Autodesk Inventor part; units mm, degrees
(part 2 of 3)
  spline S19 degree 4 poles (63.2685, 70.0081) (62.9924, 70.1512) (62.9774, 70.3018) (63.4893, 70.4674) (66.6514, 70.9944) (71.9063, 71.3106) (74.9329, 71.4009) (78.0798, 71.4009) (79.706, 71.3859) (80.218, 71.3859) (80.6245, 70.9643) (81.1365, 70.1662) (81.5129, 69.5639) (81.5975, 68.8428) knots 1 1 1 1 1 2 3 4 5 6 7 8 9 10 11 11 11 11 11
  line L530 (83.8243, 70.3846) -> (83.4753, 70.6213) construction
  line L531 (83.4753, 70.6213) -> (83.5043, 70.8246) construction
  line L532 (83.5043, 70.8246) -> (83.9543, 70.8826) construction
  line L533 (83.9543, 70.8826) -> (85.6239, 70.9407) construction
  line L534 (85.6239, 70.9407) -> (88.3822, 70.4181) construction
  line L535 (88.3822, 70.4181) -> (91.8016, 69.5461) construction
  line L536 (91.8016, 69.5461) -> (94.4571, 68.9806) construction
  line L537 (94.4571, 68.9806) -> (97.6535, 67.7512) construction
  line L538 (97.6535, 67.7512) -> (99.3008, 67.0382) construction
  line L539 (99.3008, 67.0382) -> (99.4975, 66.7677) construction
  line L540 (99.4975, 66.7677) -> (99.2517, 65.3908) construction
  line L541 (99.2517, 65.3908) -> (98.9566, 63.1533) construction
  line L542 (98.9566, 63.1533) -> (99.0304, 62.3911) construction
  line L543 (99.0304, 62.3911) -> (98.6616, 62.4649) construction
  line L544 (98.6616, 62.4649) -> (97.7272, 63.1041) construction
  line L545 (97.7272, 63.1041) -> (96.2766, 64.3581) construction
  line L546 (96.2766, 64.3581) -> (94.6292, 65.6121) construction
  line L547 (94.6292, 65.6121) -> (93.7194, 66.3497) construction
  line L548 (93.7194, 66.3497) -> (93.1539, 66.7185) construction
  line L549 (93.1539, 66.7185) -> (91.6786, 66.2022) construction
  line L550 (91.6786, 66.2022) -> (91.064, 64.8499) construction
  line L551 (91.064, 64.8499) -> (90.8673, 64.0139) construction
  line L552 (90.8673, 64.0139) -> (91.359, 62.9074) construction
  line L553 (91.359, 62.9074) -> (91.9491, 61.5551) construction
  line L554 (91.9491, 61.5551) -> (92.0596, 61.2579) construction
  line L555 (92.0596, 61.2579) -> (92.1675, 61.1272) construction
  spline S20 degree 4 poles (83.8243, 70.3846) (83.4753, 70.6213) (83.5043, 70.8246) (83.9543, 70.8826) (85.6239, 70.9407) (88.3822, 70.4181) (91.8016, 69.5461) (94.4571, 68.9806) (97.6535, 67.7512) (99.3008, 67.0382) (99.4975, 66.7677) (99.2517, 65.3908) (98.9566, 63.1533) (99.0304, 62.3911) (98.6616, 62.4649) (97.7272, 63.1041) (96.2766, 64.3581) (94.6292, 65.6121) (93.7194, 66.3497) (93.1539, 66.7185) (91.6786, 66.2022) (91.064, 64.8499) (90.8673, 64.0139) (91.359, 62.9074) (91.9491, 61.5551) (92.0596, 61.2579) (92.1675, 61.1272) knots 1 1 1 1 1 2 3 4 5 6 7 8 9 10 11 12 13 14 15 16 17 18 19 20 21 22 23 24 24 24 24 24
  line L556 (92.0596, 60.9567) -> (90.2836, 60.8762) construction
  line L557 (90.2836, 60.8762) -> (89.3753, 60.8573) construction
  line L558 (89.3753, 60.8573) -> (87.0288, 60.6113) construction
  line L559 (87.0288, 60.6113) -> (85.6286, 60.6491) construction
  line L560 (85.6286, 60.6491) -> (84.6446, 60.5923) construction
  line L561 (84.6446, 60.5923) -> (84.7203, 59.684) construction
  line L562 (84.7203, 59.684) -> (84.4932, 59.1921) construction
  line L563 (84.4932, 59.1921) -> (83.9066, 59.211) construction
  line L564 (83.9066, 59.211) -> (82.7523, 59.4948) construction
  line L565 (82.7523, 59.4948) -> (81.2763, 59.8733) construction
  line L566 (81.2763, 59.8733) -> (78.1729, 60.0814) construction
  line L567 (78.1729, 60.0814) -> (74.5776, 60.0625) construction
  line L568 (74.5776, 60.0625) -> (70.7362, 60.1382) construction
  line L569 (70.7362, 60.1382) -> (68.1817, 60.0625) construction
  line L570 (68.1817, 60.0625) -> (65.7974, 60.0057) construction
  line L571 (65.7974, 60.0057) -> (62.3156, 59.4759) construction
  line L572 (62.3156, 59.4759) -> (59.761, 58.7758) construction
  line L573 (59.761, 58.7758) -> (57.3956, 58.1702) construction
  line L574 (57.3956, 58.1702) -> (56.7712, 57.9053) construction
  line L575 (56.7712, 57.9053) -> (56.8847, 57.0916) construction
  line L576 (56.8847, 57.0916) -> (57.2064, 56.4104) construction
  line L577 (57.2064, 56.4104) -> (58.9284, 56.2022) construction
  line L578 (58.9284, 56.2022) -> (61.1234, 55.9373) construction
  line L579 (61.1234, 55.9373) -> (63.5266, 55.4832) construction
  line L580 (63.5266, 55.4832) -> (65.0594, 55.1047) construction
  line L581 (65.0594, 55.1047) -> (65.3354, 54.7866) construction
  spline S21 degree 4 poles (92.0596, 60.9567) (90.2836, 60.8762) (89.3753, 60.8573) (87.0288, 60.6113) (85.6286, 60.6491) (84.6446, 60.5923) (84.7203, 59.684) (84.4932, 59.1921) (83.9066, 59.211) (82.7523, 59.4948) (81.2763, 59.8733) (78.1729, 60.0814) (74.5776, 60.0625) (70.7362, 60.1382) (68.1817, 60.0625) (65.7974, 60.0057) (62.3156, 59.4759) (59.761, 58.7758) (57.3956, 58.1702) (56.7712, 57.9053) (56.8847, 57.0916) (57.2064, 56.4104) (58.9284, 56.2022) (61.1234, 55.9373) (63.5266, 55.4832) (65.0594, 55.1047) (65.3354, 54.7866) knots 1 1 1 1 1 2 3 4 5 6 7 8 9 10 11 12 13 14 15 16 17 18 19 20 21 22 23 24 24 24 24 24
  line L582 (65.4191, 54.3358) -> (65.081, 53.9607) construction
  line L583 (65.081, 53.9607) -> (63.7918, 52.863) construction
  line L584 (63.7918, 52.863) -> (62.9342, 51.842) construction
  line L585 (62.9342, 51.842) -> (61.7906, 50.5759) construction
  line L586 (61.7906, 50.5759) -> (61.0351, 49.269) construction
  line L587 (61.0351, 49.269) -> (60.2182, 48.2888) construction
  line L588 (60.2182, 48.2888) -> (59.4831, 46.5326) construction
  line L589 (59.4831, 46.5326) -> (59.1155, 45.144) construction
  line L590 (59.1155, 45.144) -> (58.6459, 43.4696) construction
  line L591 (58.6459, 43.4696) -> (58.217, 41.6113) construction
  line L592 (58.217, 41.6113) -> (58.0128, 38.9975) construction
  line L593 (58.0128, 38.9975) -> (57.9924, 37.4659) construction
  line L594 (57.9924, 37.4659) -> (57.8131, 36.3636) construction
  spline S22 degree 4 poles (65.4191, 54.3358) (65.081, 53.9607) (63.7918, 52.863) (62.9342, 51.842) (61.7906, 50.5759) (61.0351, 49.269) (60.2182, 48.2888) (59.4831, 46.5326) (59.1155, 45.144) (58.6459, 43.4696) (58.217, 41.6113) (58.0128, 38.9975) (57.9924, 37.4659) (57.8131, 36.3636) knots 1 1 1 1 1 2 3 4 5 6 7 8 9 10 11 11 11 11 11
  line L595 (8.3598, 43.6237) -> (9.8064, 44.3371) construction
  line L596 (9.8064, 44.3371) -> (11.9481, 45.3894) construction
  line L597 (11.9481, 45.3894) -> (15.3774, 46.6645) construction
  line L598 (15.3774, 46.6645) -> (20.0406, 48.2611) construction
  line L599 (20.0406, 48.2611) -> (24.339, 49.7917) construction
  line L600 (24.339, 49.7917) -> (29.2664, 51.3853) construction
  line L601 (29.2664, 51.3853) -> (32.9147, 52.5385) construction
  line L602 (32.9147, 52.5385) -> (36.626, 53.524) construction
  line L603 (36.626, 53.524) -> (38.6389, 54.174) construction
  line L604 (38.6389, 54.174) -> (40.6099, 54.174) construction
  line L605 (40.6099, 54.174) -> (43.5034, 53.2723) construction
  line L606 (43.5034, 53.2723) -> (46.2292, 52.9788) construction
  line L607 (46.2292, 52.9788) -> (48.934, 52.853) construction
  line L608 (48.934, 52.853) -> (51.5759, 52.6643) construction
  line L609 (51.5759, 52.6643) -> (52.6732, 52.6191) construction
  line L610 (52.6732, 52.6191) -> (53.2041, 52.6249) construction
  line L611 (53.2041, 52.6249) -> (53.245, 52.409) construction
  line L612 (53.245, 52.409) -> (52.8832, 51.8547) construction
  line L613 (52.8832, 51.8547) -> (51.8388, 50.6003) construction
  line L614 (51.8388, 50.6003) -> (50.5853, 48.4878) construction
  line L615 (50.5853, 48.4878) -> (49.3133, 45.3915) construction
  line L616 (49.3133, 45.3915) -> (48.2924, 42.3454) construction
  line L617 (48.2924, 42.3454) -> (47.9242, 40.2365) construction
  line L618 (47.9242, 40.2365) -> (48.192, 39.5168) construction
  line L619 (48.192, 39.5168) -> (48.8112, 38.9478) construction
  line L620 (48.8112, 38.9478) -> (48.51, 38.5126) construction
  line L621 (48.51, 38.5126) -> (48.0915, 37.3578) construction
  line L622 (48.0915, 37.3578) -> (48.0078, 36.3535) construction
  line L623 (48.0078, 36.3535) -> (48.7108, 34.6129) construction
  line L624 (48.7108, 34.6129) -> (49.6313, 32.4036) construction
  line L625 (49.6313, 32.4036) -> (50.8364, 30.0939) construction
  line L626 (50.8364, 30.0939) -> (52.008, 28.6546) construction
  line L627 (52.008, 28.6546) -> (54.3177, 26.0771) construction
  line L628 (54.3177, 26.0771) -> (55.9411, 24.6879) construction
  line L629 (55.9411, 24.6879) -> (57.2466, 24.1858) construction
  line L630 (57.2466, 24.1858) -> (57.7487, 24.3364) construction
  line L631 (57.7487, 24.3364) -> (58.4851, 24.4201) construction
  line L632 (58.4851, 24.4201) -> (58.865, 24.189) construction
  line L633 (58.865, 24.189) -> (58.95, 23.1685) construction
  line L634 (58.95, 23.1685) -> (59.8855, 22.2898) construction
  line L635 (59.8855, 22.2898) -> (62.465, 21.2409) construction
  line L636 (62.465, 21.2409) -> (65.5265, 20.5889) construction
  line L637 (65.5265, 20.5889) -> (70.7139, 20.0504) construction
  line L638 (70.7139, 20.0504) -> (74.4557, 19.937) construction
  line L639 (74.4557, 19.937) -> (76.8368, 20.0504) construction
  line L640 (76.8368, 20.0504) -> (78.3912, 20.0214) construction
  line L641 (78.3912, 20.0214) -> (78.6619, 19.922) construction
  spline S23 degree 4 poles (8.3598, 43.6237) (9.8064, 44.3371) (11.9481, 45.3894) (15.3774, 46.6645) (20.0406, 48.2611) (24.339, 49.7917) (29.2664, 51.3853) (32.9147, 52.5385) (36.626, 53.524) (38.6389, 54.174) (40.6099, 54.174) (43.5034, 53.2723) (46.2292, 52.9788) (48.934, 52.853) (51.5759, 52.6643) (52.6732, 52.6191) (53.2041, 52.6249) (53.245, 52.409) (52.8832, 51.8547) (51.8388, 50.6003) (50.5853, 48.4878) (49.3133, 45.3915) (48.2924, 42.3454) (47.9242, 40.2365) (48.192, 39.5168) (48.8112, 38.9478) (48.51, 38.5126) (48.0915, 37.3578) (48.0078, 36.3535) (48.7108, 34.6129) (49.6313, 32.4036) (50.8364, 30.0939) (52.008, 28.6546) (54.3177, 26.0771) (55.9411, 24.6879) (57.2466, 24.1858) (57.7487, 24.3364) (58.4851, 24.4201) (58.865, 24.189) (58.95, 23.1685) (59.8855, 22.2898) (62.465, 21.2409) (65.5265, 20.5889) (70.7139, 20.0504) (74.4557, 19.937) (76.8368, 20.0504) (78.3912, 20.0214) (78.6619, 19.922) knots 1 1 1 1 1 2 3 4 5 6 7 8 9 10 11 12 13 14 15 16 17 18 19 20 21 22 23 24 25 26 27 28 29 30 31 32 33 34 35 36 37 38 39 40 41 42 43 44 45 45 45 45 45
  line L642 (65.081, 28.397) -> (65.0019, 29.199) construction
  line L643 (65.0019, 29.199) -> (65.2705, 30.0048) construction
  line L644 (65.2705, 30.0048) -> (65.4415, 30.9327) construction
  line L645 (65.4415, 30.9327) -> (64.9043, 31.9338) construction
  line L646 (64.9043, 31.9338) -> (64.831, 33.4477) construction
  line L647 (64.831, 33.4477) -> (64.8066, 36.0849) construction
  line L648 (64.8066, 36.0849) -> (65.2217, 38.3313) construction
  line L649 (65.2217, 38.3313) -> (65.881, 39.4545) construction
  line L650 (65.881, 39.4545) -> (66.0763, 40.0162) construction
  line L651 (66.0763, 40.0162) -> (65.9054, 40.1383) construction
  line L652 (65.9054, 40.1383) -> (65.5265, 40.0607) construction
  line L653 (65.5265, 40.0607) -> (65.4932, 40.0607) construction
  spline S24 degree 4 poles (65.081, 28.397) (65.0019, 29.199) (65.2705, 30.0048) (65.4415, 30.9327) (64.9043, 31.9338) (64.831, 33.4477) (64.8066, 36.0849) (65.2217, 38.3313) (65.881, 39.4545) (66.0763, 40.0162) (65.9054, 40.1383) (65.5265, 40.0607) (65.4932, 40.0607) knots 1 1 1 1 1 2 3 4 5 6 7 8 9 10 10 10 10 10
  line L654 (52.8179, 63.6057) -> (51.2391, 63.3355) construction
  line L655 (51.2391, 63.3355) -> (49.1343, 62.8712) construction
  line L656 (49.1343, 62.8712) -> (46.2247, 62.6546) construction
  line L657 (46.2247, 62.6546) -> (43.9342, 63.676) construction
  line L658 (43.9342, 63.676) -> (42.4794, 64.1713) construction
  line L659 (42.4794, 64.1713) -> (43.7175, 63.0879) construction
  line L660 (43.7175, 63.0879) -> (46.2557, 61.726) construction
  line L661 (46.2557, 61.726) -> (47.0295, 61.3545) construction
  line L662 (47.0295, 61.3545) -> (49.2581, 61.6641) construction
  line L663 (49.2581, 61.6641) -> (51.6725, 61.695) construction
  line L664 (51.6725, 61.695) -> (53.5606, 62.1903) construction
  line L665 (53.5606, 62.1903) -> (54.5202, 62.9022) construction
  line L666 (54.5202, 62.9022) -> (58.2346, 64.7594) construction
  line L667 (58.2346, 64.7594) -> (59.256, 65.3475) construction
  line L668 (59.256, 65.3475) -> (58.5558, 65.9056) construction
  line L669 (58.5558, 65.9056) -> (57.07, 66.4008) construction
  line L670 (57.07, 66.4008) -> (54.8104, 66.8342) construction
  line L671 (54.8104, 66.8342) -> (53.1699, 66.8961) construction
  line L672 (53.1699, 66.8961) -> (51.158, 66.927) construction
  line L673 (51.158, 66.927) -> (49.3317, 66.8342) construction
  line L674 (49.3317, 66.8342) -> (48.7746, 66.6794) construction
  line L675 (48.7746, 66.6794) -> (49.7935, 66.0783) construction
  line L676 (49.7935, 66.0783) -> (50.5932, 66.0134) construction
  line L677 (50.5932, 66.0134) -> (51.2955, 65.9403) construction
  line L678 (51.2955, 65.9403) -> (51.6297, 65.9403) construction
  spline S25 degree 4 poles (52.8179, 63.6057) (51.2391, 63.3355) (49.1343, 62.8712) (46.2247, 62.6546) (43.9342, 63.676) (42.4794, 64.1713) (43.7175, 63.0879) (46.2557, 61.726) (47.0295, 61.3545) (49.2581, 61.6641) (51.6725, 61.695) (53.5606, 62.1903) (54.5202, 62.9022) (58.2346, 64.7594) (59.256, 65.3475) (58.5558, 65.9056) (57.07, 66.4008) (54.8104, 66.8342) (53.1699, 66.8961) (51.158, 66.927) (49.3317, 66.8342) (48.7746, 66.6794) (49.7935, 66.0783) (50.5932, 66.0134) (51.2955, 65.9403) (51.6297, 65.9403) knots 1 1 1 1 1 2 3 4 5 6 7 8 9 10 11 12 13 14 15 16 17 18 19 20 21 22 23 23 23 23 23
  line L679 (66.9113, 53.2103) -> (66.1589, 52.2511) construction
  line L680 (66.1589, 52.2511) -> (64.5343, 50.6524) construction
  line L681 (64.5343, 50.6524) -> (62.9548, 48.7893) construction
  line L682 (62.9548, 48.7893) -> (61.517, 46.5415) construction
  line L683 (61.517, 46.5415) -> (60.8892, 45.2657) construction
  line L684 (60.8892, 45.2657) -> (60.8082, 44.1924) construction
  line L685 (60.8082, 44.1924) -> (61.1322, 44.3342) construction
  line L686 (61.1322, 44.3342) -> (61.4562, 44.6987) construction
  line L687 (61.4562, 44.6987) -> (62.2865, 45.9745) construction
  line L688 (62.2865, 45.9745) -> (63.6028, 47.6958) construction
  line L689 (63.6028, 47.6958) -> (65.1014, 49.1538) construction
  line L690 (65.1014, 49.1538) -> (66.9644, 50.7739) construction
  line L691 (66.9644, 50.7739) -> (69.273, 52.3534) construction
  line L692 (69.273, 52.3534) -> (70.5083, 53.1432) construction
  line L693 (70.5083, 53.1432) -> (72.0878, 53.6292) construction
  line L694 (72.0878, 53.6292) -> (72.7359, 54.095) construction
  line L695 (72.7359, 54.095) -> (71.9056, 54.3988) construction
  line L696 (71.9056, 54.3988) -> (70.002, 55.067) construction
  line L697 (70.002, 55.067) -> (68.9895, 55.5935) construction
  line L698 (68.9895, 55.5935) -> (68.6524, 55.7505) construction
  line L699 (68.6524, 55.7505) -> (68.4709, 55.5789) construction
  spline S26 degree 4 poles (66.9113, 53.2103) (66.1589, 52.2511) (64.5343, 50.6524) (62.9548, 48.7893) (61.517, 46.5415) (60.8892, 45.2657) (60.8082, 44.1924) (61.1322, 44.3342) (61.4562, 44.6987) (62.2865, 45.9745) (63.6028, 47.6958) (65.1014, 49.1538) (66.9644, 50.7739) (69.273, 52.3534) (70.5083, 53.1432) (72.0878, 53.6292) (72.7359, 54.095) (71.9056, 54.3988) (70.002, 55.067) (68.9895, 55.5935) (68.6524, 55.7505) (68.4709, 55.5789) knots 1 1 1 1 1 2 3 4 5 6 7 8 9 10 11 12 13 14 15 16 17 18 19 19 19 19 19
  line L700 (66.3059, 56.3646) -> (65.6237, 56.9327) construction
  line L701 (65.6237, 56.9327) -> (64.7343, 56.992) construction
  line L702 (64.7343, 56.992) -> (64.1414, 57.1698) construction
  line L703 (64.1414, 57.1698) -> (64.3192, 57.5256) construction
  line L704 (64.3192, 57.5256) -> (65.3074, 57.7627) construction
  line L705 (65.3074, 57.7627) -> (67.8965, 58.0592) construction
  line L706 (67.8965, 58.0592) -> (72.9955, 58.2568) construction
  line L707 (72.9955, 58.2568) -> (78.8851, 58.158) construction
  line L708 (78.8851, 58.158) -> (82.6204, 57.5058) construction
  line L709 (82.6204, 57.5058) -> (87.0277, 56.7548) construction
  line L710 (87.0277, 56.7548) -> (91.5734, 55.1935) construction
  line L711 (91.5734, 55.1935) -> (95.5261, 53.2369) construction
  line L712 (95.5261, 53.2369) -> (94.9728, 53.1776) construction
  line L713 (94.9728, 53.1776) -> (90.3283, 54.7389) construction
  line L714 (90.3283, 54.7389) -> (86.0593, 55.905) construction
  line L715 (86.0593, 55.905) -> (83.747, 56.4979) construction
  line L716 (83.747, 56.4979) -> (81.8694, 56.4583) construction
  line L717 (81.8694, 56.4583) -> (81.1777, 56.5572) construction
  line L718 (81.1777, 56.5572) -> (80.6836, 57.071) construction
  line L719 (80.6836, 57.071) -> (79.7942, 57.4465) construction
  line L720 (79.7942, 57.4465) -> (75.9008, 57.5849) construction
  line L721 (75.9008, 57.5849) -> (72.5212, 57.5849) construction
  line L722 (72.5212, 57.5849) -> (68.9044, 57.5453) construction
  line L723 (68.9044, 57.5453) -> (68.2522, 57.2884) construction
  line L724 (68.2522, 57.2884) -> (68.2522, 56.6362) construction
  line L725 (68.2522, 56.6362) -> (68.0022, 56.4202) construction
  line L726 (68.0022, 56.4202) -> (67.7877, 56.3707) construction
  line L727 (67.7877, 56.3707) -> (67.6792, 56.3575) construction
  spline S27 degree 4 poles (66.3059, 56.3646) (65.6237, 56.9327) (64.7343, 56.992) (64.1414, 57.1698) (64.3192, 57.5256) (65.3074, 57.7627) (67.8965, 58.0592) (72.9955, 58.2568) (78.8851, 58.158) (82.6204, 57.5058) (87.0277, 56.7548) (91.5734, 55.1935) (95.5261, 53.2369) (94.9728, 53.1776) (90.3283, 54.7389) (86.0593, 55.905) (83.747, 56.4979) (81.8694, 56.4583) (81.1777, 56.5572) (80.6836, 57.071) (79.7942, 57.4465) (75.9008, 57.5849) (72.5212, 57.5849) (68.9044, 57.5453) (68.2522, 57.2884) (68.2522, 56.6362) (68.0022, 56.4202) (67.7877, 56.3707) (67.6792, 56.3575) knots 1 1 1 1 1 2 3 4 5 6 7 8 9 10 11 12 13 14 15 16 17 18 19 20 21 22 23 24 25 26 26 26 26 26
  line L728 (83.5333, 54.3147) -> (83.6608, 54.5518) construction
  line L729 (83.6608, 54.5518) -> (84.3663, 54.6016) construction
  line L730 (84.3663, 54.6016) -> (85.7855, 54.1285) construction
  line L731 (85.7855, 54.1285) -> (87.4123, 53.6804) construction
  line L732 (87.4123, 53.6804) -> (88.9477, 53.2737) construction
  line L733 (88.9477, 53.2737) -> (89.7196, 53.0164) construction
  line L734 (89.7196, 53.0164) -> (88.8066, 52.9002) construction
  line L735 (88.8066, 52.9002) -> (87.3625, 52.8089) construction
  line L736 (87.3625, 52.8089) -> (86.3831, 52.3939) construction
  line L737 (86.3831, 52.3939) -> (85.4535, 52.2445) construction
  line L738 (85.4535, 52.2445) -> (84.1754, 51.788) construction
  line L739 (84.1754, 51.788) -> (83.3288, 51.6718) construction
  line L740 (83.3288, 51.6718) -> (82.4823, 51.6635) construction
  line L741 (82.4823, 51.6635) -> (82.1171, 51.2818) construction
  line L742 (82.1171, 51.2818) -> (81.6357, 51.3316) construction
  line L743 (81.6357, 51.3316) -> (81.0962, 51.6303) construction
  line L744 (81.0962, 51.6303) -> (80.7974, 51.871) construction
  line L745 (80.7974, 51.871) -> (80.5485, 52.2362) construction
  line L746 (80.5485, 52.2362) -> (80.3892, 52.409) construction
  spline S28 degree 4 poles (83.5333, 54.3147) (83.6608, 54.5518) (84.3663, 54.6016) (85.7855, 54.1285) (87.4123, 53.6804) (88.9477, 53.2737) (89.7196, 53.0164) (88.8066, 52.9002) (87.3625, 52.8089) (86.3831, 52.3939) (85.4535, 52.2445) (84.1754, 51.788) (83.3288, 51.6718) (82.4823, 51.6635) (82.1171, 51.2818) (81.6357, 51.3316) (81.0962, 51.6303) (80.7974, 51.871) (80.5485, 52.2362) (80.3892, 52.409) knots 1 1 1 1 1 2 3 4 5 6 7 8 9 10 11 12 13 14 15 16 17 17 17 17 17
  line L747 (80.6729, 54.336) -> (80.4498, 54.7426) construction
  line L748 (80.4498, 54.7426) -> (79.8635, 55.2788) construction
  line L749 (79.8635, 55.2788) -> (79.6776, 55.4718) construction
  line L750 (79.6776, 55.4718) -> (79.0985, 55.6077) construction
  line L751 (79.0985, 55.6077) -> (77.8903, 55.6148) construction
  line L752 (77.8903, 55.6148) -> (76.153, 55.6506) construction
  line L753 (76.153, 55.6506) -> (75.5239, 55.6434) construction
  line L754 (75.5239, 55.6434) -> (75.3094, 55.5362) construction
  line L755 (75.3094, 55.5362) -> (75.3094, 55.3431) construction
  line L756 (75.3094, 55.3431) -> (75.8885, 55.0429) construction
  line L757 (75.8885, 55.0429) -> (76.5176, 54.6854) construction
  line L758 (76.5176, 54.6854) -> (76.9823, 54.0777) construction
  line L759 (76.9823, 54.0777) -> (76.6606, 53.6487) construction
  line L760 (76.6606, 53.6487) -> (76.1101, 53.0053) construction
  line L761 (76.1101, 53.0053) -> (75.3594, 52.655) construction
  line L762 (75.3594, 52.655) -> (73.1404, 52.0547) construction
  line L763 (73.1404, 52.0547) -> (70.3924, 50.6397) construction
  line L764 (70.3924, 50.6397) -> (66.824, 47.9942) construction
  line L765 (66.824, 47.9942) -> (64.9783, 46.292) construction
  line L766 (64.9783, 46.292) -> (63.4812, 44.5283) construction
  line L767 (63.4812, 44.5283) -> (62.4353, 42.8262) construction
  line L768 (62.4353, 42.8262) -> (61.1023, 39.955) construction
  line L769 (61.1023, 39.955) -> (60.3435, 38.0683) construction
  line L770 (60.3435, 38.0683) -> (60.323, 36.6943) construction
  line L771 (60.323, 36.6943) -> (60.323, 36.2863) construction
  spline S29 degree 4 poles (80.6729, 54.336) (80.4498, 54.7426) (79.8635, 55.2788) (79.6776, 55.4718) (79.0985, 55.6077) (77.8903, 55.6148) (76.153, 55.6506) (75.5239, 55.6434) (75.3094, 55.5362) (75.3094, 55.3431) (75.8885, 55.0429) (76.5176, 54.6854) (76.9823, 54.0777) (76.6606, 53.6487) (76.1101, 53.0053) (75.3594, 52.655) (73.1404, 52.0547) (70.3924, 50.6397) (66.824, 47.9942) (64.9783, 46.292) (63.4812, 44.5283) (62.4353, 42.8262) (61.1023, 39.955) (60.3435, 38.0683) (60.323, 36.6943) (60.323, 36.2863) knots 1 1 1 1 1 2 3 4 5 6 7 8 9 10 11 12 13 14 15 16 17 18 19 20 21 22 23 23 23 23 23
  line L772 (94.0312, 61.726) -> (93.7051, 62.2473) construction
  line L773 (93.7051, 62.2473) -> (93.1799, 63.181) construction
  line L774 (93.1799, 63.181) -> (93.1799, 63.6645) construction
  line L775 (93.1799, 63.6645) -> (93.3716, 63.8229) construction
  line L776 (93.3716, 63.8229) -> (93.7884, 63.5811) construction
  line L777 (93.7884, 63.5811) -> (94.7138, 62.9726) construction
  line L778 (94.7138, 62.9726) -> (95.7475, 62.1889) construction
  line L779 (95.7475, 62.1889) -> (97.198, 61.1469) construction
  line L780 (97.198, 61.1469) -> (97.9081, 60.597) construction
  spline S30 degree 4 poles (94.0312, 61.726) (93.7051, 62.2473) (93.1799, 63.181) (93.1799, 63.6645) (93.3716, 63.8229) (93.7884, 63.5811) (94.7138, 62.9726) (95.7475, 62.1889) (97.198, 61.1469) (97.9081, 60.597) knots 1 1 1 1 1 2 3 4 5 6 7 7 7 7 7
  line L781 (92.326, 59.0061) -> (91.721, 59.1295) construction
  line L782 (91.721, 59.1295) -> (90.1871, 59.2295) construction
  line L783 (90.1871, 59.2295) -> (89.1701, 59.2545) construction
  line L784 (89.1701, 59.2545) -> (88.1864, 59.2295) construction
  line L785 (88.1864, 59.2295) -> (87.9697, 58.9461) construction
  line L786 (87.9697, 58.9461) -> (87.9697, 58.6627) construction
  line L787 (87.9697, 58.6627) -> (87.9863, 58.4376) construction
  line L788 (87.9863, 58.4376) -> (88.4448, 58.1208) construction
  line L789 (88.4448, 58.1208) -> (90.5289, 57.5039) construction
  line L790 (90.5289, 57.5039) -> (92.513, 56.7286) construction
  line L791 (92.513, 56.7286) -> (95.2528, 55.6483) construction
  line L792 (95.2528, 55.6483) -> (98.4333, 53.807) construction
  line L793 (98.4333, 53.807) -> (102.1876, 51.6787) construction
  line L794 (102.1876, 51.6787) -> (103.8615, 50.0766) construction
  line L795 (103.8615, 50.0766) -> (105.1289, 49.3113) construction
  line L796 (105.1289, 49.3113) -> (106.0551, 49.0264) construction
  spline S31 degree 4 poles (92.326, 59.0061) (91.721, 59.1295) (90.1871, 59.2295) (89.1701, 59.2545) (88.1864, 59.2295) (87.9697, 58.9461) (87.9697, 58.6627) (87.9863, 58.4376) (88.4448, 58.1208) (90.5289, 57.5039) (92.513, 56.7286) (95.2528, 55.6483) (98.4333, 53.807) (102.1876, 51.6787) (103.8615, 50.0766) (105.1289, 49.3113) (106.0551, 49.0264) knots 1 1 1 1 1 2 3 4 5 6 7 8 9 10 11 12 13 14 14 14 14 14
  line L797 (104.2741, 46.5328) -> (103.7785, 46.9222) construction
  line L798 (103.7785, 46.9222) -> (102.9329, 47.282) construction
  line L799 (102.9329, 47.282) -> (102.3571, 47.309) construction
  line L800 (102.3571, 47.309) -> (101.6014, 47.291) construction
  line L801 (101.6014, 47.291) -> (101.4395, 47.0571) construction
  line L802 (101.4395, 47.0571) -> (100.9627, 46.6163) construction
  line L803 (100.9627, 46.6163) -> (99.9012, 46.0315) construction
  line L804 (99.9012, 46.0315) -> (99.0106, 45.6177) construction
  line L805 (99.0106, 45.6177) -> (97.931, 45.6537) construction
  line L806 (97.931, 45.6537) -> (96.6626, 45.9056) construction
  line L807 (96.6626, 45.9056) -> (95.61, 46.1305) construction
  line L808 (95.61, 46.1305) -> (94.3955, 46.2834) construction
  line L809 (94.3955, 46.2834) -> (93.2081, 46.5533) construction
  line L810 (93.2081, 46.5533) -> (92.3714, 46.5983) construction
  line L811 (92.3714, 46.5983) -> (91.9396, 46.6703) construction
  line L812 (91.9396, 46.6703) -> (91.5977, 46.4094) construction
  line L813 (91.5977, 46.4094) -> (91.022, 45.7707) construction
  line L814 (91.022, 45.7707) -> (90.5182, 45.2399) construction
  line L815 (90.5182, 45.2399) -> (90.0144, 44.7001) construction
  line L816 (90.0144, 44.7001) -> (89.4837, 44.3583) construction
  line L817 (89.4837, 44.3583) -> (88.638, 43.9624) construction
  line L818 (88.638, 43.9624) -> (88.0803, 43.9354) construction
  line L819 (88.0803, 43.9354) -> (87.5135, 43.9264) construction
  line L820 (87.5135, 43.9264) -> (87.0997, 43.8995) construction
  line L821 (87.0997, 43.8995) -> (86.7938, 43.5036) construction
  line L822 (86.7938, 43.5036) -> (86.2181, 42.721) construction
  line L823 (86.2181, 42.721) -> (85.9932, 42.2262) construction
  line L824 (85.9932, 42.2262) -> (85.5434, 41.6684) construction
  line L825 (85.5434, 41.6684) -> (85.1295, 41.2906) construction
  line L826 (85.1295, 41.2906) -> (84.3829, 40.9127) construction
  line L827 (84.3829, 40.9127) -> (83.3521, 40.3324) construction
  line L828 (83.3521, 40.3324) -> (82.4075, 39.1897) construction
  line L829 (82.4075, 39.1897) -> (81.8437, 38.1536) construction
  line L830 (81.8437, 38.1536) -> (81.4323, 37.2699) construction
  line L831 (81.4323, 37.2699) -> (81.4476, 36.3709) construction
  line L832 (81.4476, 36.3709) -> (81.3866, 35.6396) construction
  line L833 (81.3866, 35.6396) -> (81.6761, 35.1215) construction
  line L834 (81.6761, 35.1215) -> (81.8894, 34.7558) construction
  line L835 (81.8894, 34.7558) -> (82.3618, 34.0093) construction
  line L836 (82.3618, 34.0093) -> (83.0626, 33.1103) construction
  line L837 (83.0626, 33.1103) -> (83.2536, 32.9024) construction
  spline S32 degree 4 poles (104.2741, 46.5328) (103.7785, 46.9222) (102.9329, 47.282) (102.3571, 47.309) (101.6014, 47.291) (101.4395, 47.0571) (100.9627, 46.6163) (99.9012, 46.0315) (99.0106, 45.6177) (97.931, 45.6537) (96.6626, 45.9056) (95.61, 46.1305) (94.3955, 46.2834) (93.2081, 46.5533) (92.3714, 46.5983) (91.9396, 46.6703) (91.5977, 46.4094) (91.022, 45.7707) (90.5182, 45.2399) (90.0144, 44.7001) (89.4837, 44.3583) (88.638, 43.9624) (88.0803, 43.9354) (87.5135, 43.9264) (87.0997, 43.8995) (86.7938, 43.5036) (86.2181, 42.721) (85.9932, 42.2262) (85.5434, 41.6684) (85.1295, 41.2906) (84.3829, 40.9127) (83.3521, 40.3324) (82.4075, 39.1897) (81.8437, 38.1536) (81.4323, 37.2699) (81.4476, 36.3709) (81.3866, 35.6396) (81.6761, 35.1215) (81.8894, 34.7558) (82.3618, 34.0093) (83.0626, 33.1103) (83.2536, 32.9024) knots 1 1 1 1 1 2 3 4 5 6 7 8 9 10 11 12 13 14 15 16 17 18 19 20 21 22 23 24 25 26 27 28 29 30 31 32 33 34 35 36 37 38 39 39 39 39 39
  line L838 (65.9903, 42.721) -> (66.2881, 42.6424) construction
  line L839 (66.2881, 42.6424) -> (67.6606, 42.7681) construction
  line L840 (67.6606, 42.7681) -> (68.6873, 43.3757) construction
  line L841 (68.6873, 43.3757) -> (70.2797, 45.0101) construction
  line L842 (70.2797, 45.0101) -> (71.9035, 46.2672) construction
  line L843 (71.9035, 46.2672) -> (72.9093, 46.8958) construction
  line L844 (72.9093, 46.8958) -> (75.057, 48.132) construction
  line L845 (75.057, 48.132) -> (76.157, 48.9702) construction
  line L846 (76.157, 48.9702) -> (77.7285, 49.7454) construction
  line L847 (77.7285, 49.7454) -> (78.7656, 50.0597) construction
  line L848 (78.7656, 50.0597) -> (78.9434, 50.2021) construction
  spline S33 degree 4 poles (65.9903, 42.721) (66.2881, 42.6424) (67.6606, 42.7681) (68.6873, 43.3757) (70.2797, 45.0101) (71.9035, 46.2672) (72.9093, 46.8958) (75.057, 48.132) (76.157, 48.9702) (77.7285, 49.7454) (78.7656, 50.0597) (78.9434, 50.2021) knots 1 1 1 1 1 2 3 4 5 6 7 8 9 9 9 9 9
  line L849 (83.6268, 31.2422) -> (83.1411, 31.1284) construction
  line L850 (83.1411, 31.1284) -> (82.0253, 31.3729) construction
  line L851 (82.0253, 31.3729) -> (81.2611, 32.3664) construction
  line L852 (81.2611, 32.3664) -> (80.3898, 33.9101) construction
  line L853 (80.3898, 33.9101) -> (79.5951, 35.729) construction
  line L854 (79.5951, 35.729) -> (79.702, 36.967) construction
  line L855 (79.702, 36.967) -> (79.8855, 37.6854) construction
  line L856 (79.8855, 37.6854) -> (80.5427, 39.382) construction
  line L857 (80.5427, 39.382) -> (81.4292, 40.6965) construction
  line L858 (81.4292, 40.6965) -> (82.0864, 41.1397) construction
  line L859 (82.0864, 41.1397) -> (82.4227, 41.7969) construction
  line L860 (82.4227, 41.7969) -> (82.1934, 41.9192) construction
  line L861 (82.1934, 41.9192) -> (81.796, 41.7664) construction
  line L862 (81.796, 41.7664) -> (80.7567, 40.8799) construction
  line L863 (80.7567, 40.8799) -> (79.8702, 39.5501) construction
  line L864 (79.8702, 39.5501) -> (79.0907, 37.9911) construction
  line L865 (79.0907, 37.9911) -> (78.9073, 36.3251) construction
  line L866 (78.9073, 36.3251) -> (79.702, 33.849) construction
  line L867 (79.702, 33.849) -> (80.0994, 33.0084) construction
  line L868 (80.0994, 33.0084) -> (80.879, 31.5563) construction
  line L869 (80.879, 31.5563) -> (82.117, 30.2266) construction
  line L870 (82.117, 30.2266) -> (84.0428, 28.7593) construction
  line L871 (84.0428, 28.7593) -> (84.7918, 28.3619) construction
  line L872 (84.7918, 28.3619) -> (84.9829, 28.4041) construction
  spline S34 degree 4 poles (83.6268, 31.2422) (83.1411, 31.1284) (82.0253, 31.3729) (81.2611, 32.3664) (80.3898, 33.9101) (79.5951, 35.729) (79.702, 36.967) (79.8855, 37.6854) (80.5427, 39.382) (81.4292, 40.6965) (82.0864, 41.1397) (82.4227, 41.7969) (82.1934, 41.9192) (81.796, 41.7664) (80.7567, 40.8799) (79.8702, 39.5501) (79.0907, 37.9911) (78.9073, 36.3251) (79.702, 33.849) (80.0994, 33.0084) (80.879, 31.5563) (82.117, 30.2266) (84.0428, 28.7593) (84.7918, 28.3619) (84.9829, 28.4041) knots 1 1 1 1 1 2 3 4 5 6 7 8 9 10 11 12 13 14 15 16 17 18 19 20 21 22 22 22 22 22
  line L873 (85.2963, 26.5309) -> (84.6565, 26.5488) construction
  line L874 (84.6565, 26.5488) -> (83.5658, 27.0287) construction
  line L875 (83.5658, 27.0287) -> (81.6171, 28.6284) construction
  line L876 (81.6171, 28.6284) -> (79.6392, 30.7372) construction
  line L877 (79.6392, 30.7372) -> (79.1738, 31.4789) construction
  line L878 (79.1738, 31.4789) -> (78.1704, 33.5585) construction
  line L879 (78.1704, 33.5585) -> (77.5014, 34.911) construction
  line L880 (77.5014, 34.911) -> (77.3851, 36.7289) construction
  line L881 (77.3851, 36.7289) -> (77.5887, 38.8085) construction
  line L882 (77.5887, 38.8085) -> (78.0686, 40.1465) construction
  line L883 (78.0686, 40.1465) -> (79.1738, 41.6153) construction
  line L884 (79.1738, 41.6153) -> (80.3373, 42.4297) construction
  line L885 (80.3373, 42.4297) -> (81.4716, 43.3895) construction
  line L886 (81.4716, 43.3895) -> (83.7258, 44.3639) construction
  line L887 (83.7258, 44.3639) -> (85.8054, 45.1638) construction
  line L888 (85.8054, 45.1638) -> (87.9723, 45.6146) construction
  line L889 (87.9723, 45.6146) -> (88.2486, 45.8473) construction
  line L890 (88.2486, 45.8473) -> (88.1759, 46.0509) construction
  line L891 (88.1759, 46.0509) -> (87.6669, 46.1818) construction
  line L892 (87.6669, 46.1818) -> (86.5326, 46.0364) construction
  line L893 (86.5326, 46.0364) -> (83.7258, 45.2365) construction
  line L894 (83.7258, 45.2365) -> (81.1808, 43.9713) construction
  line L895 (81.1808, 43.9713) -> (79.1448, 42.6333) construction
  line L896 (79.1448, 42.6333) -> (77.865, 40.9172) construction
  line L897 (77.865, 40.9172) -> (77.036, 38.8521) construction
  line L898 (77.036, 38.8521) -> (76.6143, 36.1035) construction
  line L899 (76.6143, 36.1035) -> (76.687, 35.1291) construction
  line L900 (76.687, 35.1291) -> (77.2396, 33.6312) construction
  line L901 (77.2396, 33.6312) -> (78.4467, 31.5807) construction
  line L902 (78.4467, 31.5807) -> (79.9446, 29.5592) construction
  line L903 (79.9446, 29.5592) -> (82.2569, 27.2759) construction
  line L904 (82.2569, 27.2759) -> (85.5291, 25.1672) construction
  line L905 (85.5291, 25.1672) -> (88.1323, 23.4657) construction
  line L906 (88.1323, 23.4657) -> (88.8449, 23.3057) construction
  line L907 (88.8449, 23.3057) -> (89.6448, 23.9311) construction
  line L908 (89.6448, 23.9311) -> (89.8629, 24.4692) construction
  line L909 (89.8629, 24.4692) -> (89.5284, 25.0654) construction
  line L910 (89.5284, 25.0654) -> (89.1212, 25.9235) construction
  line L911 (89.1212, 25.9235) -> (88.7286, 27.3777) construction
  line L912 (88.7286, 27.3777) -> (89.034, 28.803) construction
  line L913 (89.034, 28.803) -> (89.543, 30.8826) construction
  line L914 (89.543, 30.8826) -> (92.052, 33.5775) construction
  line L915 (92.052, 33.5775) -> (94.4542, 35.9091) construction
  line L916 (94.4542, 35.9091) -> (96.2912, 37.1102) construction
  line L917 (96.2912, 37.1102) -> (97.9163, 38.382) construction
  line L918 (97.9163, 38.382) -> (98.9018, 39.2124) construction
  line L919 (98.9018, 39.2124) -> (98.9804, 39.5663) construction
  line L920 (98.9804, 39.5663) -> (98.4496, 39.6253) construction
  line L921 (98.4496, 39.6253) -> (97.7088, 39.6605) construction
  spline S35 degree 4 poles (85.2963, 26.5309) (84.6565, 26.5488) (83.5658, 27.0287) (81.6171, 28.6284) (79.6392, 30.7372) (79.1738, 31.4789) (78.1704, 33.5585) (77.5014, 34.911) (77.3851, 36.7289) (77.5887, 38.8085) (78.0686, 40.1465) (79.1738, 41.6153) (80.3373, 42.4297) (81.4716, 43.3895) (83.7258, 44.3639) (85.8054, 45.1638) (87.9723, 45.6146) (88.2486, 45.8473) (88.1759, 46.0509) (87.6669, 46.1818) (86.5326, 46.0364) (83.7258, 45.2365) (81.1808, 43.9713) (79.1448, 42.6333) (77.865, 40.9172) (77.036, 38.8521) (76.6143, 36.1035) (76.687, 35.1291) (77.2396, 33.6312) (78.4467, 31.5807) (79.9446, 29.5592) (82.2569, 27.2759) (85.5291, 25.1672) (88.1323, 23.4657) (88.8449, 23.3057) (89.6448, 23.9311) (89.8629, 24.4692) (89.5284, 25.0654) (89.1212, 25.9235) (88.7286, 27.3777) (89.034, 28.803) (89.543, 30.8826) (92.052, 33.5775) (94.4542, 35.9091) (96.2912, 37.1102) (97.9163, 38.382) (98.9018, 39.2124) (98.9804, 39.5663) (98.4496, 39.6253) (97.7088, 39.6605) knots 1 1 1 1 1 2 3 4 5 6 7 8 9 10 11 12 13 14 15 16 17 18 19 20 21 22 23 24 25 26 27 28 29 30 31 32 33 34 35 36 37 38 39 40 41 42 43 44 45 46 47 47 47 47 47
  line L922 (92.4223, 23.1183) -> (91.3149, 22.9284) construction
  line L923 (91.3149, 22.9284) -> (90.7425, 22.0354) construction
  line L924 (90.7425, 22.0354) -> (89.8496, 21.2798) construction
  line L925 (89.8496, 21.2798) -> (87.995, 21.3485) construction
  line L926 (87.995, 21.3485) -> (86.5983, 22.2415) construction
  line L927 (86.5983, 22.2415) -> (82.5227, 24.8288) construction
  line L928 (82.5227, 24.8288) -> (80.1186, 26.7979) construction
  line L929 (80.1186, 26.7979) -> (77.7145, 29.4767) construction
  line L930 (77.7145, 29.4767) -> (76.3407, 31.629) construction
  line L931 (76.3407, 31.629) -> (75.6538, 32.8196) construction
  line L932 (75.6538, 32.8196) -> (75.1501, 34.4911) construction
  line L933 (75.1501, 34.4911) -> (75.0356, 35.2924) construction
  line L934 (75.0356, 35.2924) -> (75.0814, 36.712) construction
  line L935 (75.0814, 36.712) -> (75.2417, 38.1087) construction
  line L936 (75.2417, 38.1087) -> (75.9057, 40.7647) construction
  line L937 (75.9057, 40.7647) -> (76.7528, 41.9324) construction
  line L938 (76.7528, 41.9324) -> (79.4682, 44.6822) construction
  line L939 (79.4682, 44.6822) -> (80.4376, 45.2638) construction
  line L940 (80.4376, 45.2638) -> (82.0663, 45.9231) construction
  line L941 (82.0663, 45.9231) -> (82.6093, 46.3109) construction
  line L942 (82.6093, 46.3109) -> (84.5094, 46.9701) construction
  line L943 (84.5094, 46.9701) -> (85.8667, 47.5906) construction
  line L944 (85.8667, 47.5906) -> (87.1464, 47.7845) construction
  line L945 (87.1464, 47.7845) -> (88.969, 47.9784) construction
  line L946 (88.969, 47.9784) -> (91.1018, 48.1335) construction
  line L947 (91.1018, 48.1335) -> (94.7083, 47.9784) construction
  line L948 (94.7083, 47.9784) -> (97.9269, 47.5518) construction
  line L949 (97.9269, 47.5518) -> (98.6359, 47.7101) construction
  line L950 (98.6359, 47.7101) -> (98.6701, 47.9662) construction
  line L951 (98.6701, 47.9662) -> (97.8276, 48.3191) construction
  line L952 (97.8276, 48.3191) -> (95.545, 48.6095) construction
  line L953 (95.545, 48.6095) -> (92.0015, 48.6561) construction
  line L954 (92.0015, 48.6561) -> (88.1851, 48.5455) construction
  line L955 (88.1851, 48.5455) -> (85.2259, 48.1306) construction
  line L956 (85.2259, 48.1306) -> (81.7966, 46.5819) construction
  line L957 (81.7966, 46.5819) -> (79.114, 45.2268) construction
  line L958 (79.114, 45.2268) -> (77.0398, 43.3185) construction
  line L959 (77.0398, 43.3185) -> (75.0486, 40.3041) construction
  line L960 (75.0486, 40.3041) -> (74.1913, 37.7874) construction
  line L961 (74.1913, 37.7874) -> (74.3019, 34.7176) construction
  line L962 (74.3019, 34.7176) -> (74.5231, 33.3348) construction
  line L963 (74.5231, 33.3348) -> (76.3208, 30.2927) construction
  line L964 (76.3208, 30.2927) -> (79.031, 26.974) construction
  line L965 (79.031, 26.974) -> (80.9116, 25.5083) construction
  line L966 (80.9116, 25.5083) -> (85.2812, 22.0236) construction
  line L967 (85.2812, 22.0236) -> (89.0977, 20.226) construction
  line L968 (89.0977, 20.226) -> (92.1398, 18.0412) construction
  line L969 (92.1398, 18.0412) -> (93.0248, 16.6308) construction
  line L970 (93.0248, 16.6308) -> (94.6012, 15.4692) construction
  line L971 (94.6012, 15.4692) -> (97.0625, 14.5566) construction
  line L972 (97.0625, 14.5566) -> (100.0494, 13.0079) construction
  line L973 (100.0494, 13.0079) -> (104.1147, 11.4868) construction
  line L974 (104.1147, 11.4868) -> (105.1735, 11.8091) construction
  spline S36 degree 4 poles (92.4223, 23.1183) (91.3149, 22.9284) (90.7425, 22.0354) (89.8496, 21.2798) (87.995, 21.3485) (86.5983, 22.2415) (82.5227, 24.8288) (80.1186, 26.7979) (77.7145, 29.4767) (76.3407, 31.629) (75.6538, 32.8196) (75.1501, 34.4911) (75.0356, 35.2924) (75.0814, 36.712) (75.2417, 38.1087) (75.9057, 40.7647) (76.7528, 41.9324) (79.4682, 44.6822) (80.4376, 45.2638) (82.0663, 45.9231) (82.6093, 46.3109) (84.5094, 46.9701) (85.8667, 47.5906) (87.1464, 47.7845) (88.969, 47.9784) (91.1018, 48.1335) (94.7083, 47.9784) (97.9269, 47.5518) (98.6359, 47.7101) (98.6701, 47.9662) (97.8276, 48.3191) (95.545, 48.6095) (92.0015, 48.6561) (88.1851, 48.5455) (85.2259, 48.1306) (81.7966, 46.5819) (79.114, 45.2268) (77.0398, 43.3185) (75.0486, 40.3041) (74.1913, 37.7874) (74.3019, 34.7176) (74.5231, 33.3348) (76.3208, 30.2927) (79.031, 26.974) (80.9116, 25.5083) (85.2812, 22.0236) (89.0977, 20.226) (92.1398, 18.0412) (93.0248, 16.6308) (94.6012, 15.4692) (97.0625, 14.5566) (100.0494, 13.0079) (104.1147, 11.4868) (105.1735, 11.8091) knots 1 1 1 1 1 2 3 4 5 6 7 8 9 10 11 12 13 14 15 16 17 18 19 20 21 22 23 24 25 26 27 28 29 30 31 32 33 34 35 36 37 38 39 40 41 42 43 44 45 46 47 48 49 50 51 51 51 51 51
  line L975 (106.2958, 14.2226) -> (106.8369, 13.7198) construction
  line L976 (106.8369, 13.7198) -> (107.7005, 13.7718) construction
  line L977 (107.7005, 13.7718) -> (108.127, 13.9903) construction
  line L978 (108.127, 13.9903) -> (108.8241, 14.7706) construction
  line L979 (108.8241, 14.7706) -> (110.4576, 17.7774) construction
  line L980 (110.4576, 17.7774) -> (110.8945, 18.8698) construction
  line L981 (110.8945, 18.8698) -> (111.0298, 19.4837) construction
  line L982 (111.0298, 19.4837) -> (111.0728, 19.6578) construction
  spline S37 degree 4 poles (106.2958, 14.2226) (106.8369, 13.7198) (107.7005, 13.7718) (108.127, 13.9903) (108.8241, 14.7706) (110.4576, 17.7774) (110.8945, 18.8698) (111.0298, 19.4837) (111.0728, 19.6578) knots 1 1 1 1 1 2 3 4 5 6 6 6 6 6
  line L983 (110.836, 20.5889) -> (110.4159, 20.805) construction
  line L984 (110.4159, 20.805) -> (110.0102, 21.5125) construction
  line L985 (110.0102, 21.5125) -> (110.0102, 21.9391) construction
  line L986 (110.0102, 21.9391) -> (110.4472, 22.272) construction
  line L987 (110.4472, 22.272) -> (111.165, 22.8859) construction
  line L988 (111.165, 22.8859) -> (111.8227, 23.9268) construction
  line L989 (111.8227, 23.9268) -> (113.4665, 25.2847) construction
  line L990 (113.4665, 25.2847) -> (116.1823, 27.8813) construction
  line L991 (116.1823, 27.8813) -> (118.231, 30.3113) construction
  line L992 (118.231, 30.3113) -> (118.9219, 31.7168) construction
  line L993 (118.9219, 31.7168) -> (119.0886, 32.6697) construction
  line L994 (119.0886, 32.6697) -> (118.6837, 33.575) construction
  line L995 (118.6837, 33.575) -> (118.3025, 34.1705) construction
  line L996 (118.3025, 34.1705) -> (117.1114, 34.5755) construction
  line L997 (117.1114, 34.5755) -> (115.1341, 35.1711) construction
  line L998 (115.1341, 35.1711) -> (113.5618, 35.6714) construction
  line L999 (113.5618, 35.6714) -> (113.2283, 35.5284) construction
  line L1000 (113.2283, 35.5284) -> (114.1812, 34.8614) construction
  line L1001 (114.1812, 34.8614) -> (115.4438, 33.575) construction
  line L1002 (115.4438, 33.575) -> (116.0155, 31.1212) construction
  line L1003 (116.0155, 31.1212) -> (115.4914, 29.0487) construction
  line L1004 (115.4914, 29.0487) -> (113.7285, 27.2381) construction
  line L1005 (113.7285, 27.2381) -> (111.4416, 24.8559) construction
  line L1006 (111.4416, 24.8559) -> (109.1784, 23.2597) construction
  line L1007 (109.1784, 23.2597) -> (107.4155, 21.8304) construction
  line L1008 (107.4155, 21.8304) -> (106.1291, 21.0681) construction
  line L1009 (106.1291, 21.0681) -> (105.1286, 20.806) construction
  line L1010 (105.1286, 20.806) -> (104.3186, 20.9966) construction
  line L1011 (104.3186, 20.9966) -> (103.2704, 21.3778) construction
  line L1012 (103.2704, 21.3778) -> (101.8887, 21.9257) construction
  line L1013 (101.8887, 21.9257) -> (101.1263, 21.9495) construction
  line L1014 (101.1263, 21.9495) -> (100.9088, 21.8735) construction
  spline S38 degree 4 poles (110.836, 20.5889) (110.4159, 20.805) (110.0102, 21.5125) (110.0102, 21.9391) (110.4472, 22.272) (111.165, 22.8859) (111.8227, 23.9268) (113.4665, 25.2847) (116.1823, 27.8813) (118.231, 30.3113) (118.9219, 31.7168) (119.0886, 32.6697) (118.6837, 33.575) (118.3025, 34.1705) (117.1114, 34.5755) (115.1341, 35.1711) (113.5618, 35.6714) (113.2283, 35.5284) (114.1812, 34.8614) (115.4438, 33.575) (116.0155, 31.1212) (115.4914, 29.0487) (113.7285, 27.2381) (111.4416, 24.8559) (109.1784, 23.2597) (107.4155, 21.8304) (106.1291, 21.0681) (105.1286, 20.806) (104.3186, 20.9966) (103.2704, 21.3778) (101.8887, 21.9257) (101.1263, 21.9495) (100.9088, 21.8735) knots 1 1 1 1 1 2 3 4 5 6 7 8 9 10 11 12 13 14 15 16 17 18 19 20 21 22 23 24 25 26 27 28 29 30 30 30 30 30
  line L1015 (101.564, 23.7452) -> (102.3866, 23.4432) construction
  line L1016 (102.3866, 23.4432) -> (103.8469, 23.0112) construction
  line L1017 (103.8469, 23.0112) -> (104.9789, 22.7519) construction
  line L1018 (104.9789, 22.7519) -> (105.3504, 22.8643) construction
  line L1019 (105.3504, 22.8643) -> (105.2554, 23.1667) construction
  line L1020 (105.2554, 23.1667) -> (104.9097, 23.4691) construction
  line L1021 (104.9097, 23.4691) -> (104.2012, 23.7629) construction
  line L1022 (104.2012, 23.7629) -> (102.81, 24.3505) construction
  line L1023 (102.81, 24.3505) -> (101.0214, 24.8171) construction
  line L1024 (101.0214, 24.8171) -> (99.9153, 25.0245) construction
  line L1025 (99.9153, 25.0245) -> (98.0575, 25.3269) construction
  line L1026 (98.0575, 25.3269) -> (95.8282, 25.3442) construction
  line L1027 (95.8282, 25.3442) -> (95.3357, 25.4565) construction
  line L1028 (95.3357, 25.4565) -> (95.0169, 25.5156) construction
  spline S39 degree 4 poles (101.564, 23.7452) (102.3866, 23.4432) (103.8469, 23.0112) (104.9789, 22.7519) (105.3504, 22.8643) (105.2554, 23.1667) (104.9097, 23.4691) (104.2012, 23.7629) (102.81, 24.3505) (101.0214, 24.8171) (99.9153, 25.0245) (98.0575, 25.3269) (95.8282, 25.3442) (95.3357, 25.4565) (95.0169, 25.5156) knots 1 1 1 1 1 2 3 4 5 6 7 8 9 10 11 12 12 12 12 12
  line L1029 (98.8062, 42.0604) -> (99.5157, 41.3809) construction
  line L1030 (99.5157, 41.3809) -> (101.4159, 41.1461) construction
  line L1031 (101.4159, 41.1461) -> (102.9532, 41.445) construction
  line L1032 (102.9532, 41.445) -> (104.3624, 41.7653) construction
  line L1033 (104.3624, 41.7653) -> (106.4761, 41.9147) construction
  line L1034 (106.4761, 41.9147) -> (107.4796, 42.235) construction
  line L1035 (107.4796, 42.235) -> (109.4866, 41.9788) construction
  line L1036 (109.4866, 41.9788) -> (111.3505, 41.6684) construction
  line L1037 (111.3505, 41.6684) -> (112.4421, 41.9788) construction
  line L1038 (112.4421, 41.9788) -> (112.7874, 42.6333) construction
  line L1039 (112.7874, 42.6333) -> (112.9758, 42.6333) construction
  spline S40 degree 4 poles (98.8062, 42.0604) (99.5157, 41.3809) (101.4159, 41.1461) (102.9532, 41.445) (104.3624, 41.7653) (106.4761, 41.9147) (107.4796, 42.235) (109.4866, 41.9788) (111.3505, 41.6684) (112.4421, 41.9788) (112.7874, 42.6333) (112.9758, 42.6333) knots 1 1 1 1 1 2 3 4 5 6 7 8 9 9 9 9 9
  line L1040 (115.0822, 43.7015) -> (115.0931, 42.6796) construction
  line L1041 (115.0931, 42.6796) -> (115.061, 42.1218) construction
  line L1042 (115.061, 42.1218) -> (115.3047, 41.5063) construction
  line L1043 (115.3047, 41.5063) -> (115.8304, 41.019) construction
  line L1044 (115.8304, 41.019) -> (117.3469, 40.4976) construction
  line L1045 (117.3469, 40.4976) -> (119.3094, 39.3763) construction
  line L1046 (119.3094, 39.3763) -> (121.7702, 37.7253) construction
  line L1047 (121.7702, 37.7253) -> (123.2031, 36.2924) construction
  line L1048 (123.2031, 36.2924) -> (124.1687, 35.4514) construction
  line L1049 (124.1687, 35.4514) -> (124.5011, 35.1949) construction
  spline S41 degree 4 poles (115.0822, 43.7015) (115.0931, 42.6796) (115.061, 42.1218) (115.3047, 41.5063) (115.8304, 41.019) (117.3469, 40.4976) (119.3094, 39.3763) (121.7702, 37.7253) (123.2031, 36.2924) (124.1687, 35.4514) (124.5011, 35.1949) knots 1 1 1 1 1 2 3 4 5 6 7 8 8 8 8 8
  line L1050 (124.6795, 35.1711) -> (125.2026, 35.4494) construction
  line L1051 (125.2026, 35.4494) -> (125.324, 35.7875) construction
  line L1052 (125.324, 35.7875) -> (125.168, 36.1428) construction
  line L1053 (125.168, 36.1428) -> (125.0726, 36.7843) construction
  line L1054 (125.0726, 36.7843) -> (125.2373, 37.391) construction
  line L1055 (125.2373, 37.391) -> (125.9394, 38.1625) construction
  line L1056 (125.9394, 38.1625) -> (126.8149, 39.2113) construction
  line L1057 (126.8149, 39.2113) -> (127.6932, 39.9851) construction
  line L1058 (127.6932, 39.9851) -> (127.7311, 40.1884) construction
  line L1059 (127.7311, 40.1884) -> (127.6435, 40.2371) construction
  line L1060 (127.6435, 40.2371) -> (127.5896, 40.3185) construction
  spline S42 degree 4 poles (124.6795, 35.1711) (125.2026, 35.4494) (125.324, 35.7875) (125.168, 36.1428) (125.0726, 36.7843) (125.2373, 37.391) (125.9394, 38.1625) (126.8149, 39.2113) (127.6932, 39.9851) (127.7311, 40.1884) (127.6435, 40.2371) (127.5896, 40.3185) knots 1 1 1 1 1 2 3 4 5 6 7 8 9 9 9 9 9
  line L1061 (128.7603, 42.3454) -> (128.8456, 42.8245) construction
  line L1062 (128.8456, 42.8245) -> (128.6763, 43.5273) construction
  line L1063 (128.6763, 43.5273) -> (128.1258, 44.3911) construction
  line L1064 (128.1258, 44.3911) -> (127.0842, 45.3227) construction
  line L1065 (127.0842, 45.3227) -> (125.2126, 46.7623) construction
  line L1066 (125.2126, 46.7623) -> (123.1463, 48.5322) construction
  line L1067 (123.1463, 48.5322) -> (122.037, 49.794) construction
  line L1068 (122.037, 49.794) -> (121.7744, 49.7094) construction
  line L1069 (121.7744, 49.7094) -> (121.3764, 49.3283) construction
  line L1070 (121.3764, 49.3283) -> (120.8481, 49.2126) construction
  spline S43 degree 4 poles (128.7603, 42.3454) (128.8456, 42.8245) (128.6763, 43.5273) (128.1258, 44.3911) (127.0842, 45.3227) (125.2126, 46.7623) (123.1463, 48.5322) (122.037, 49.794) (121.7744, 49.7094) (121.3764, 49.3283) (120.8481, 49.2126) knots 1 1 1 1 1 2 3 4 5 6 7 8 8 8 8 8
  line L1071 (121.3764, 52.0329) -> (122.5555, 51.423) construction
  line L1072 (122.5555, 51.423) -> (124.3304, 50.7304) construction
  line L1073 (124.3304, 50.7304) -> (126.2568, 50.2109) construction
  line L1074 (126.2568, 50.2109) -> (128.0317, 49.7347) construction
  line L1075 (128.0317, 49.7347) -> (128.1688, 49.8533) construction
  line L1076 (128.1688, 49.8533) -> (128.3423, 50.0879) construction
  line L1077 (128.3423, 50.0879) -> (127.9036, 50.6184) construction
  line L1078 (127.9036, 50.6184) -> (126.5366, 52.0058) construction